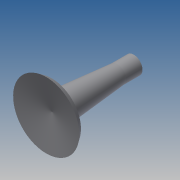
# Autodesk Inventor part: Robot1_B_Ventouse
Saved by Autodesk Inventor 2015 SP1 (Build 190203100, 203)
## iProperties
Created: 2014-10-26
Part Number: Robot1_B_Ventouse
Material: Generic
Document SubType Name: Modeling
Designer: Flopy
Density: 1 g/cm^3
Appearance: Default
Author: Flopy
Autodesk Inventor part; units mm, degrees
ref_plane "YZ Plane" through (0, 0, 0) normal (1, 0, 0) x (0, 1, 0)
ref_plane "XZ Plane" through (0, 0, 0) normal (0, 1, 0) x (-1, 0, 0)
ref_plane "XY Plane" through (0, 0, 0) normal (0, 0, 1) x (1, 0, 0)
sketch "Sketch1" plane through (0, 0, 0) normal (1, 0, 0) x (0, 1, 0)
  line L0 (0, -11.3426) -> (1.9174, -10)
  line L1 (1.9174, -10) -> (4.3655, -4.75)
  line L2 (4.3655, -4.75) -> (24.3681, -3)
  line L3 (24.3681, -3) -> (30, -3)
  line L4 (30, -3) -> (30, 0)
  line L5 (30, 0) -> (2, 0)
  line L6 (2, 0) -> (0, -11.3426)
  point P0 (0, 0)
  dimension "d0" = 30
  dimension "d2" = 20
  dimension "d3" = 6
  dimension "d4" = 5
  dimension "d5" = 100
  dimension "d6" = 2
  dimension "d7" = 45
  dimension "d8" = 15
  dimension "d9" = 9.5
  constraints: 14 end point, 2 perpendicular, 1 horizontal, 1 point on line, 1 vertical alignment
  measures "d0" distance from line of L4 point (0, 0)
  measures "d2" diameter of L0.end L5
  measures "d3" diameter of L3 L5
  measures "d4" angle of L3 L2
  measures "d5" angle of L5 L6
  measures "d6" distance of point (0, 0) L5.end
  measures "d7" angle of L6 L0
  measures "d8" angle of L1 L6
  measures "d9" diameter of L1.end L5
revolve "Revolution1" add sketch "Sketch1" angle 360 about axis through (0, 30, 0) along (0, -1, 0)
body "Solid1"
